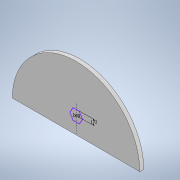
# Autodesk Inventor part: Rear
Saved by Autodesk Inventor 2021 (Build 250183000, 183)
## iProperties
Created: 2021-03-27
Part Number: Rear
Material: Generic
Document SubType Name: Modeling
Designer: cmzgt
Density: 1 g/cm^3
Appearance: Default
Author: cmzgt
Autodesk Inventor part; units mm, degrees
ref_plane "YZ Plane" through (0, 0, 0) normal (1, 0, 0) x (0, 1, 0)
ref_plane "XZ Plane" through (0, 0, 0) normal (0, 1, 0) x (-1, 0, 0)
ref_plane "XY Plane" through (0, 0, 0) normal (0, 0, 1) x (1, 0, 0)
sketch "Sketch1" plane through (0, 0, 0) normal (0, 0, 1) x (1, 0, 0)
  arc A0 (50.8, 0) -> (-50.8, 0) centre (0, 0) ccw
  line L0 (0, 0) -> (50.8, 0)
  line L1 (0, 0) -> (-50.8, 0)
  dimension "d0" = 101.6
  constraints: 4 end point, 2 horizontal, 2 point on circle, 1 centre point, 1 coincident
  measures "d0" diameter of A0
extrude "Extrusion1" add sketch "Sketch1" along normal blind 3.175
sketch "Sketch4" plane through (0, 0, 0) normal (0, 0, -1) x (-1, 0, 0)
  line L0 (0, 0) -> (0, 12.7) construction
  line L1 (0, 12.7) -> (12.7, 12.7) construction
  circle A0 centre (12.7, 12.7) radius 3.175
  circle A1 centre (-12.7, 12.7) radius 3.175
  dimension "d15" = 12.7
  dimension "d16" = 12.7
  dimension "d17" = 6.35
  constraints: 4 end point, 2 centre point, 1 coincident, 1 perpendicular, 1 symmetric about line, 1 vertical, 1 other
  measures "d15" distance of L0.start L0.end
  measures "d16" distance of L0.end L1.end
  measures "d17" diameter of A0
extrude "Extrusion5" add sketch "Sketch4" along normal blind 19.05
sketch "Sketch5" plane through (0, 0, 3.175) normal (0, 0, 1) x (1, 0, 0)
  line L0 (-2.5936, 17.577) -> (2.4467, 17.6618)
  line L1 (2.4467, 17.6618) -> (5.0403, 13.3391)
  line L2 (5.0403, 13.3391) -> (2.5936, 8.9317)
  line L3 (2.5936, 8.9317) -> (-2.4467, 8.8469)
  line L4 (-2.4467, 8.8469) -> (-5.0403, 13.1696)
  line L5 (-5.0403, 13.1696) -> (-2.5936, 17.577)
  line L6 (0, 0) -> (0, 21.7215) construction
  point P0 (0, 13.2543)
  dimension "d22" = 4.3656
  dimension "d23" = 0
  constraints: 14 end point, 1 vertical, 13 other
  measures "d22" distance from line of point (0, 13.254) L0
  measures "d23" distance from line of L6 point (0, 13.254)
body "Solid1"
